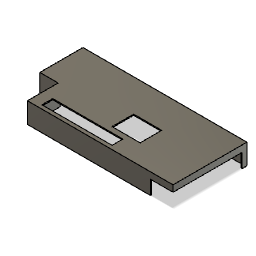
GeigerCounterTop v2 (Autodesk Fusion 360 design; units mm, degrees)
Autodesk Fusion 360 part; units mm, degrees
sketch "Skizze1" plane through (0, 0, 0) normal (0, 1, 0) x (1, 0, 0)
  line L0 (0, 0) -> (135, 0)
  line L1 (135, 0) -> (135, -68.5)
  line L2 (135, -68.5) -> (0, -68.5)
  line L3 (0, -68.5) -> (0, 0)
  dimension "d1" = 135
  dimension "d2" = 68.5
  constraint horizontal L0
  constraint vertical L1
  constraint horizontal L2
  constraint vertical L3
  constraint coincident L0.start L3.end
  measures "d1" distance of L0.start L0.end
  measures "d2" distance of L0.start L2.end
extrude "Extrusion1" add sketch "Skizze1" along normal blind 1
sketch "Skizze2" plane through (0, 0, 0) normal (0, 1, 0) x (1, 0, 0)
  line L0 (0, 0) -> (-17, 0)
  line L1 (-17, 0) -> (-17, -40)
  line L2 (-17, -40) -> (0, -40)
  line L3 (0, -40) -> (0, 0)
  dimension "d5" = 17
  dimension "d6" = 40
  constraint horizontal L0
  constraint vertical L1
  constraint horizontal L2
  constraint vertical L3
  constraint coincident L0.start L3.end
  measures "d5" distance of L0.start L0.end
  measures "d6" distance of L0.start L2.end
extrude "Extrusion2" add sketch "Skizze2" along normal blind 1
sketch "Skizze3" plane through (0, 1, 0) normal (0, 1, 0) x (-1, 0, 0)
  line L0 (0, 68.5) -> (-135, 68.5)
  line L1 (-135, 68.5) -> (-135, 0)
  line L2 (-135, 0) -> (17, 0)
  line L3 (17, 0) -> (17, 40)
  line L4 (17, 40) -> (0, 40)
  line L5 (0, 40) -> (0, 68.5)
  line L6 (-10, 65) -> (-75, 65)
  line L7 (-75, 65) -> (-75, 55)
  line L8 (-75, 55) -> (-10, 55)
  line L9 (-10, 55) -> (-10, 65)
  dimension "d9" = 65
  dimension "d10" = 10
  constraint horizontal L6
  constraint vertical L7
  constraint horizontal L8
  constraint vertical L9
  measures "d9" distance of L6.start L6.end
  measures "d10" distance of L6.start L8.end
extrude "Extrusion3" cut sketch "Skizze3" against normal blind 1 contours L6 L7 L8 L9
sketch "Skizze4" plane through (0, 1, 0) normal (0, 1, 0) x (-1, 0, 0)
  line L0 (-75, 65) -> (-10, 65)
  line L1 (-10, 65) -> (-10, 55)
  line L2 (-10, 55) -> (-75, 55)
  line L3 (-75, 55) -> (-75, 65)
  line L4 (0, 68.5) -> (-135, 68.5)
  line L5 (-135, 68.5) -> (-135, 0)
  line L6 (-135, 0) -> (17, 0)
  line L7 (17, 0) -> (17, 40)
  line L8 (17, 40) -> (0, 40)
  line L9 (0, 40) -> (0, 68.5)
  line L10 (-60, 50) -> (-86, 50)
  line L11 (-86, 50) -> (-86, 30)
  line L12 (-86, 30) -> (-60, 30)
  line L13 (-60, 30) -> (-60, 50)
  dimension "d13" = 26
  dimension "d14" = 20
  constraint horizontal L10
  constraint vertical L11
  constraint horizontal L12
  constraint vertical L13
  measures "d13" distance of L10.start L10.end
  measures "d14" distance of L10.start L12.end
extrude "Extrusion4" cut sketch "Skizze4" against normal blind 1 contours L10 L11 L12 L13
sketch "Skizze5" plane through (0, 0, 0) normal (0, -1, 0) x (1, 0, 0)
  line L0 (60, 50) -> (86, 50)
  line L1 (86, 50) -> (86, 30)
  line L2 (86, 30) -> (60, 30)
  line L3 (60, 30) -> (60, 50)
  line L4 (10, 65) -> (75, 65)
  line L5 (75, 65) -> (75, 55)
  line L6 (75, 55) -> (10, 55)
  line L7 (10, 55) -> (10, 65)
  line L8 (135, 68.5) -> (0, 68.5)
  line L9 (0, 68.5) -> (0, 40)
  line L10 (0, 40) -> (-17, 40)
  line L11 (-17, 40) -> (-17, 0)
  line L12 (-17, 0) -> (135, 0)
  line L13 (135, 0) -> (135, 68.5)
  line L14 (135, 0) -> (-17, 0)
  line L15 (-17, 0) -> (-17, 0.5)
  line L16 (-17, 0.5) -> (135, 0.5)
  line L17 (135, 0.5) -> (135, 0)
  dimension "d17" = 0.5
  constraint horizontal L14
  constraint vertical L15
  constraint horizontal L16
  constraint vertical L17
  constraint coincident L12.end L13.start
  measures "d17" distance of L12.end L16.end
extrude "Extrusion5" add sketch "Skizze5" along normal blind 18 contours L11 L12 L13 L14 L15 L16 L17
sketch "Skizze6" plane through (0, 0, 0) normal (0, -1, 0) x (1, 0, 0)
  line L0 (-17, 0.5) -> (135, 0.5)
  line L1 (135, 0.5) -> (135, 68.5)
  line L2 (135, 68.5) -> (0, 68.5)
  line L3 (0, 68.5) -> (0, 40)
  line L4 (0, 40) -> (-17, 40)
  line L5 (-17, 40) -> (-17, 0.5)
  line L6 (10, 65) -> (75, 65)
  line L7 (75, 65) -> (75, 55)
  line L8 (75, 55) -> (10, 55)
  line L9 (10, 55) -> (10, 65)
  line L10 (60, 50) -> (86, 50)
  line L11 (86, 50) -> (86, 30)
  line L12 (86, 30) -> (60, 30)
  line L13 (60, 30) -> (60, 50)
  line L14 (-17, 40) -> (-16.5, 40)
  line L15 (-16.5, 40) -> (-16.5, 0.5)
  line L16 (-16.5, 0.5) -> (-17, 0.5)
  line L17 (-17, 0.5) -> (-17, 40)
  constraint horizontal L14
  constraint vertical L15
  constraint horizontal L16
  constraint vertical L17
  constraint coincident L0 L15.end
  constraint coincident L4.end L5.start
extrude "Extrusion6" add sketch "Skizze6" along normal blind 18 contours L0 L4 L5 L14 L15 L16 L17
sketch "Skizze7" plane through (0, 0, 0) normal (0, -1, 0) x (1, 0, 0)
  line L0 (60, 50) -> (86, 50)
  line L1 (86, 50) -> (86, 30)
  line L2 (86, 30) -> (60, 30)
  line L3 (60, 30) -> (60, 50)
  line L4 (10, 65) -> (75, 65)
  line L5 (75, 65) -> (75, 55)
  line L6 (75, 55) -> (10, 55)
  line L7 (10, 55) -> (10, 65)
  line L8 (-16.5, 40) -> (-16.5, 0.5)
  line L9 (-16.5, 0.5) -> (135, 0.5)
  line L10 (135, 0.5) -> (135, 68.5)
  line L11 (135, 68.5) -> (0, 68.5)
  line L12 (0, 68.5) -> (0, 40)
  line L13 (0, 40) -> (-16.5, 40)
  line L14 (0, 40) -> (-16.5, 40)
  line L15 (-16.5, 40) -> (-16.5, 39.5)
  line L16 (-16.5, 39.5) -> (0, 39.5)
  line L17 (0, 39.5) -> (0, 40)
  dimension "d22" = 0.5
  constraint horizontal L14
  constraint vertical L15
  constraint horizontal L16
  constraint vertical L17
  constraint coincident L12.end L13.start
  measures "d22" distance of L12.end L16.end
extrude "Extrusion7" add sketch "Skizze7" along normal blind 18 contours L8 L13 L14 L15 L16 L17
sketch "Skizze8" plane through (0, 0, 0) normal (0, -1, 0) x (1, 0, 0)
  line L0 (0, 40) -> (0, 39.5)
  line L1 (0, 39.5) -> (-16.5, 39.5)
  line L2 (-16.5, 39.5) -> (-16.5, 0.5)
  line L3 (-16.5, 0.5) -> (135, 0.5)
  line L4 (135, 0.5) -> (135, 68.5)
  line L5 (135, 68.5) -> (0, 68.5)
  line L6 (0, 68.5) -> (0, 40)
  line L7 (10, 65) -> (75, 65)
  line L8 (75, 65) -> (75, 55)
  line L9 (75, 55) -> (10, 55)
  line L10 (10, 55) -> (10, 65)
  line L11 (60, 50) -> (86, 50)
  line L12 (86, 50) -> (86, 30)
  line L13 (86, 30) -> (60, 30)
  line L14 (60, 30) -> (60, 50)
  line L15 (0, 68.5) -> (0.5, 68.5)
  line L16 (0.5, 68.5) -> (0.5, 39.5)
  line L17 (0.5, 39.5) -> (0, 39.5)
  line L18 (0, 39.5) -> (0, 68.5)
  constraint horizontal L15
  constraint vertical L16
  constraint horizontal L17
  constraint vertical L18
  constraint coincident L5.end L6.start
extrude "Extrusion8" add sketch "Skizze8" along normal blind 18 contours L0 L5 L6 L15 L16 L17 L18
sketch "Skizze9" plane through (0, 0, 0) normal (0, -1, 0) x (1, 0, 0)
  line L0 (60, 50) -> (86, 50)
  line L1 (86, 50) -> (86, 30)
  line L2 (86, 30) -> (60, 30)
  line L3 (60, 30) -> (60, 50)
  line L4 (10, 65) -> (75, 65)
  line L5 (75, 65) -> (75, 55)
  line L6 (75, 55) -> (10, 55)
  line L7 (10, 55) -> (10, 65)
  line L8 (0.5, 68.5) -> (0.5, 39.5)
  line L9 (0.5, 39.5) -> (-16.5, 39.5)
  line L10 (-16.5, 39.5) -> (-16.5, 0.5)
  line L11 (-16.5, 0.5) -> (135, 0.5)
  line L12 (135, 0.5) -> (135, 68.5)
  line L13 (135, 68.5) -> (0.5, 68.5)
  line L14 (0.5, 68.5) -> (114, 68.5)
  line L15 (114, 68.5) -> (114, 68)
  line L16 (114, 68) -> (0.5, 68)
  line L17 (0.5, 68) -> (0.5, 68.5)
  constraint horizontal L14
  constraint vertical L15
  constraint horizontal L16
  constraint vertical L17
  constraint coincident L8.start L13.end
extrude "Extrusion9" add sketch "Skizze9" along normal blind 18 contours L8 L13 L14 L15 L16 L17
sketch "Skizze10" plane through (0, 0, 0) normal (0, -1, 0) x (1, 0, 0)
  line L0 (114, 68.5) -> (114, 68)
  line L1 (114, 68) -> (0.5, 68)
  line L2 (0.5, 68) -> (0.5, 39.5)
  line L3 (0.5, 39.5) -> (-16.5, 39.5)
  line L4 (-16.5, 39.5) -> (-16.5, 0.5)
  line L5 (-16.5, 0.5) -> (135, 0.5)
  line L6 (135, 0.5) -> (135, 68.5)
  line L7 (135, 68.5) -> (114, 68.5)
  line L8 (10, 65) -> (75, 65)
  line L9 (75, 65) -> (75, 55)
  line L10 (75, 55) -> (10, 55)
  line L11 (10, 55) -> (10, 65)
  line L12 (60, 50) -> (86, 50)
  line L13 (86, 50) -> (86, 30)
  line L14 (86, 30) -> (60, 30)
  line L15 (60, 30) -> (60, 50)
  line L16 (135, 0.5) -> (134.5, 0.5)
  line L17 (134.5, 0.5) -> (134.5, 4.5)
  line L18 (134.5, 4.5) -> (135, 4.5)
  line L19 (135, 4.5) -> (135, 0.5)
  dimension "d29" = 0.5
  dimension "d30" = 4
  constraint horizontal L16
  constraint vertical L17
  constraint horizontal L18
  constraint vertical L19
  constraint coincident L5.end L6.start
  measures "d29" distance of L5.end L16.end
  measures "d30" distance of L5.end L18.end
extrude "Extrusion10" add sketch "Skizze10" along normal blind 18 contours L5 L6 L16 L17 L18 L19
sketch "Skizze11" plane through (0, 0, 0) normal (0, -1, 0) x (1, 0, 0)
  line L0 (60, 50) -> (86, 50)
  line L1 (86, 50) -> (86, 30)
  line L2 (86, 30) -> (60, 30)
  line L3 (60, 30) -> (60, 50)
  line L4 (10, 65) -> (75, 65)
  line L5 (75, 65) -> (75, 55)
  line L6 (75, 55) -> (10, 55)
  line L7 (10, 55) -> (10, 65)
  line L8 (134.5, 0.5) -> (134.5, 4.5)
  line L9 (134.5, 4.5) -> (135, 4.5)
  line L10 (135, 4.5) -> (135, 68.5)
  line L11 (135, 68.5) -> (114, 68.5)
  line L12 (114, 68.5) -> (114, 68)
  line L13 (114, 68) -> (0.5, 68)
  line L14 (0.5, 68) -> (0.5, 39.5)
  line L15 (0.5, 39.5) -> (-16.5, 39.5)
  line L16 (-16.5, 39.5) -> (-16.5, 0.5)
  line L17 (-16.5, 0.5) -> (134.5, 0.5)
  line L18 (135, 68.5) -> (134.5, 68.5)
  line L19 (134.5, 68.5) -> (134.5, 4.5)
  line L20 (134.5, 4.5) -> (135, 4.5)
  line L21 (135, 4.5) -> (135, 68.5)
  constraint horizontal L18
  constraint vertical L19
  constraint horizontal L20
  constraint vertical L21
  constraint coincident L8.end L9.start
  constraint coincident L10.end L11.start
extrude "Extrusion11" add sketch "Skizze11" along normal blind 5 contours L9 L10 L11 L18 L19 L20 L21
sketch "Skizze12" plane through (0, 0, 0) normal (0, -1, 0) x (1, 0, 0)
  line L0 (134.5, 0.5) -> (134.5, 68.5)
  line L1 (134.5, 68.5) -> (114, 68.5)
  line L2 (114, 68.5) -> (114, 68)
  line L3 (114, 68) -> (0.5, 68)
  line L4 (0.5, 68) -> (0.5, 39.5)
  line L5 (0.5, 39.5) -> (-16.5, 39.5)
  line L6 (-16.5, 39.5) -> (-16.5, 0.5)
  line L7 (-16.5, 0.5) -> (134.5, 0.5)
  line L8 (60, 50) -> (86, 50)
  line L9 (86, 50) -> (86, 30)
  line L10 (86, 30) -> (60, 30)
  line L11 (60, 30) -> (60, 50)
  line L12 (10, 65) -> (75, 65)
  line L13 (75, 65) -> (75, 55)
  line L14 (75, 55) -> (10, 55)
  line L15 (10, 55) -> (10, 65)
  line L16 (134.5, 68.5) -> (114, 68.5)
  line L17 (114, 68.5) -> (114, 68)
  line L18 (114, 68) -> (134.5, 68)
  line L19 (134.5, 68) -> (134.5, 68.5)
  constraint horizontal L16
  constraint vertical L17
  constraint horizontal L18
  constraint vertical L19
  constraint coincident L2.end L3.start
  constraint coincident L0.end L1.start
extrude "Extrusion12" add sketch "Skizze12" along normal blind 5 contours L0 L1 L2 L16 L17 L18 L19
sketch "Skizze13" plane through (0, 0, 0) normal (0, -1, 0) x (1, 0, 0)
  line L0 (134.5, 68) -> (0.5, 68)
  line L1 (0.5, 68) -> (0.5, 39.5)
  line L2 (0.5, 39.5) -> (-16.5, 39.5)
  line L3 (-16.5, 39.5) -> (-16.5, 0.5)
  line L4 (-16.5, 0.5) -> (134.5, 0.5)
  line L5 (134.5, 0.5) -> (134.5, 68)
  line L6 (60, 50) -> (86, 50)
  line L7 (86, 50) -> (86, 30)
  line L8 (86, 30) -> (60, 30)
  line L9 (60, 30) -> (60, 50)
  line L10 (10, 65) -> (75, 65)
  line L11 (75, 65) -> (75, 55)
  line L12 (75, 55) -> (10, 55)
  line L13 (10, 55) -> (10, 65)
  line L14 (1, 68) -> (0.5, 68)
  line L15 (0.5, 68) -> (0.5, 39.5)
  line L16 (0.5, 39.5) -> (1, 39.5)
  line L17 (1, 39.5) -> (1, 68)
  constraint horizontal L14
  constraint vertical L15
  constraint horizontal L16
  constraint vertical L17
  constraint coincident L1.end L2.start
  constraint coincident L0 L14.start
extrude "Extrusion13" add sketch "Skizze13" along normal blind 18 contours L0 L1 L14 L15 L16 L17
sketch "Skizze14" plane through (0, 0, 0) normal (0, -1, 0) x (1, 0, 0)
  line L0 (10, 65) -> (75, 65)
  line L1 (75, 65) -> (75, 55)
  line L2 (75, 55) -> (10, 55)
  line L3 (10, 55) -> (10, 65)
  line L4 (60, 50) -> (86, 50)
  line L5 (86, 50) -> (86, 30)
  line L6 (86, 30) -> (60, 30)
  line L7 (60, 30) -> (60, 50)
  line L8 (1, 68) -> (1, 39.5)
  line L9 (1, 39.5) -> (-16.5, 39.5)
  line L10 (-16.5, 39.5) -> (-16.5, 0.5)
  line L11 (-16.5, 0.5) -> (134.5, 0.5)
  line L12 (134.5, 0.5) -> (134.5, 68)
  line L13 (134.5, 68) -> (1, 68)
  line L14 (-16.5, 39) -> (1, 39)
  line L15 (1, 39) -> (1, 39.5)
  line L16 (1, 39.5) -> (-16.5, 39.5)
  line L17 (-16.5, 39.5) -> (-16.5, 39)
  constraint horizontal L14
  constraint vertical L15
  constraint horizontal L16
  constraint vertical L17
  constraint coincident L8.end L9.start
  constraint coincident L10 L14.start
extrude "Extrusion14" add sketch "Skizze14" along normal blind 18 contours L9 L10 L14 L15 L16 L17
sketch "Skizze15" plane through (0, 0, 0) normal (0, -1, 0) x (1, 0, 0)
  line L0 (1, 39) -> (-16.5, 39)
  line L1 (-16.5, 39) -> (-16.5, 0.5)
  line L2 (-16.5, 0.5) -> (134.5, 0.5)
  line L3 (134.5, 0.5) -> (134.5, 68)
  line L4 (134.5, 68) -> (1, 68)
  line L5 (1, 68) -> (1, 39)
  line L6 (10, 65) -> (75, 65)
  line L7 (75, 65) -> (75, 55)
  line L8 (75, 55) -> (10, 55)
  line L9 (10, 55) -> (10, 65)
  line L10 (60, 50) -> (86, 50)
  line L11 (86, 50) -> (86, 30)
  line L12 (86, 30) -> (60, 30)
  line L13 (60, 30) -> (60, 50)
  line L14 (-16, 39) -> (-16.5, 39)
  line L15 (-16.5, 39) -> (-16.5, 0.5)
  line L16 (-16.5, 0.5) -> (-16, 0.5)
  line L17 (-16, 0.5) -> (-16, 39)
  constraint horizontal L14
  constraint vertical L15
  constraint horizontal L16
  constraint vertical L17
  constraint coincident L1.end L2.start
  constraint coincident L0 L14.start
extrude "Extrusion15" add sketch "Skizze15" along normal blind 18 contours L0 L1 L2 L14 L15 L16 L17
sketch "Skizze16" plane through (0, 0, 0) normal (0, -1, 0) x (1, 0, 0)
  line L0 (-16, 39) -> (-16, 0.5)
  line L1 (-16, 0.5) -> (134.5, 0.5)
  line L2 (134.5, 0.5) -> (134.5, 68)
  line L3 (134.5, 68) -> (1, 68)
  line L4 (1, 68) -> (1, 39)
  line L5 (1, 39) -> (-16, 39)
  line L6 (10, 65) -> (75, 65)
  line L7 (75, 65) -> (75, 55)
  line L8 (75, 55) -> (10, 55)
  line L9 (10, 55) -> (10, 65)
  line L10 (60, 50) -> (86, 50)
  line L11 (86, 50) -> (86, 30)
  line L12 (86, 30) -> (60, 30)
  line L13 (60, 30) -> (60, 50)
  line L14 (-16, 1) -> (134.5, 1)
  line L15 (134.5, 1) -> (134.5, 0.5)
  line L16 (134.5, 0.5) -> (-16, 0.5)
  line L17 (-16, 0.5) -> (-16, 1)
  constraint horizontal L14
  constraint vertical L15
  constraint horizontal L16
  constraint vertical L17
  constraint coincident L1.end L2.start
  constraint coincident L0 L14.start
extrude "Extrusion16" add sketch "Skizze16" along normal blind 18 contours L0 L1 L2 L14 L15 L16 L17
sketch "Skizze17" plane through (0, 0, 0) normal (0, -1, 0) x (1, 0, 0)
  line L0 (-16, 1) -> (134.5, 1)
  line L1 (134.5, 1) -> (134.5, 68)
  line L2 (134.5, 68) -> (1, 68)
  line L3 (1, 68) -> (1, 39)
  line L4 (1, 39) -> (-16, 39)
  line L5 (-16, 39) -> (-16, 1)
  line L6 (10, 65) -> (75, 65)
  line L7 (75, 65) -> (75, 55)
  line L8 (75, 55) -> (10, 55)
  line L9 (10, 55) -> (10, 65)
  line L10 (60, 50) -> (86, 50)
  line L11 (86, 50) -> (86, 30)
  line L12 (86, 30) -> (60, 30)
  line L13 (60, 30) -> (60, 50)
  line L14 (114, 68) -> (1, 68)
  line L15 (1, 68) -> (1, 67.5)
  line L16 (1, 67.5) -> (114, 67.5)
  line L17 (114, 67.5) -> (114, 68)
  dimension "d45" = 0.5
  constraint horizontal L14
  constraint vertical L15
  constraint horizontal L16
  constraint vertical L17
  constraint coincident L3 L15.end
  constraint coincident L2 L14.start
  measures "d45" distance of L14.start L16.end
extrude "Extrusion17" add sketch "Skizze17" along normal blind 18 contours L2 L3 L14 L15 L16 L17
sketch "Skizze18" plane through (0, 0, 0) normal (0, -1, 0) x (1, 0, 0)
  line L0 (114, 67.5) -> (1, 67.5)
  line L1 (1, 67.5) -> (1, 39)
  line L2 (1, 39) -> (-16, 39)
  line L3 (-16, 39) -> (-16, 1)
  line L4 (-16, 1) -> (134.5, 1)
  line L5 (134.5, 1) -> (134.5, 68)
  line L6 (134.5, 68) -> (114, 68)
  line L7 (114, 68) -> (114, 67.5)
  line L8 (10, 65) -> (75, 65)
  line L9 (75, 65) -> (75, 55)
  line L10 (75, 55) -> (10, 55)
  line L11 (10, 55) -> (10, 65)
  line L12 (60, 50) -> (86, 50)
  line L13 (86, 50) -> (86, 30)
  line L14 (86, 30) -> (60, 30)
  line L15 (60, 30) -> (60, 50)
  line L16 (114, 67.5) -> (134.5, 67.5)
  line L17 (134.5, 67.5) -> (134.5, 68)
  line L18 (134.5, 68) -> (114, 68)
  line L19 (114, 68) -> (114, 67.5)
  constraint horizontal L16
  constraint vertical L17
  constraint horizontal L18
  constraint vertical L19
  constraint coincident L5.end L6.start
  constraint coincident L0.start L7.end
extrude "Extrusion18" add sketch "Skizze18" along normal blind 5 contours L5 L6 L7 L16 L17 L18 L19
sketch "Skizze19" plane through (0, 0, 0) normal (0, -1, 0) x (1, 0, 0)
  line L0 (60, 50) -> (86, 50)
  line L1 (86, 50) -> (86, 30)
  line L2 (86, 30) -> (60, 30)
  line L3 (60, 30) -> (60, 50)
  line L4 (10, 65) -> (75, 65)
  line L5 (75, 65) -> (75, 55)
  line L6 (75, 55) -> (10, 55)
  line L7 (10, 55) -> (10, 65)
  line L8 (134.5, 67.5) -> (1, 67.5)
  line L9 (1, 67.5) -> (1, 39)
  line L10 (1, 39) -> (-16, 39)
  line L11 (-16, 39) -> (-16, 1)
  line L12 (-16, 1) -> (134.5, 1)
  line L13 (134.5, 1) -> (134.5, 67.5)
  line L14 (134.5, 67.5) -> (134, 67.5)
  line L15 (134, 67.5) -> (134, 1)
  line L16 (134, 1) -> (134.5, 1)
  line L17 (134.5, 1) -> (134.5, 67.5)
  constraint horizontal L14
  constraint vertical L15
  constraint horizontal L16
  constraint vertical L17
  constraint coincident L12 L15.end
  constraint coincident L8.start L13.end
extrude "Extrusion19" add sketch "Skizze19" along normal blind 5 contours L8 L12 L13 L14 L15 L16 L17
sketch "Skizze20" plane through (0, -5, 0) normal (0, -1, 0) x (1, 0, 0)
  line L0 (135, 4.5) -> (135, 68.5)
  line L1 (135, 68.5) -> (114, 68.5)
  line L2 (114, 68.5) -> (114, 67.5)
  line L3 (114, 67.5) -> (134, 67.5)
  line L4 (134, 67.5) -> (134, 1)
  line L5 (134, 1) -> (134.5, 1)
  line L6 (134.5, 1) -> (134.5, 4.5)
  line L7 (134.5, 4.5) -> (135, 4.5)
  line L8 (134.5, 4.5) -> (134, 4.5)
  line L9 (134, 4.5) -> (134, 1)
  line L10 (134, 1) -> (134.5, 1)
  line L11 (134.5, 1) -> (134.5, 4.5)
  constraint horizontal L8
  constraint vertical L9
  constraint horizontal L10
  constraint vertical L11
  constraint coincident L4.end L5.start
  constraint coincident L6.end L7.start
extrude "Extrusion20" add sketch "Skizze20" along normal blind 13 contours L4 L5 L6 L8 L9 L10 L11
